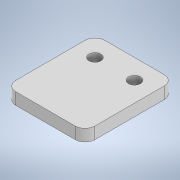
# Autodesk Inventor part: MagnetHolder_Special
Saved by Autodesk Inventor 2021 (Build 250183000, 183)
## iProperties
Created: 2021-12-05
Part Number: MagnetHolder_Special
Material: Generic
Document SubType Name: Modeling
Designer: Jorian Brusind
Density: 1 g/cm^3
Appearance: Default
Author: Jorian Brusind
Autodesk Inventor part; units mm, degrees
ref_plane "YZ Plane" through (0, 0, 0) normal (1, 0, 0) x (0, 1, 0)
ref_plane "XZ Plane" through (0, 0, 0) normal (0, 1, 0) x (-1, 0, 0)
ref_plane "XY Plane" through (0, 0, 0) normal (0, 0, 1) x (1, 0, 0)
sketch "Sketch20" plane through (0, 0, 0) normal (0, 1, 0) x (-1, 0, 0)
  line L0 (0, 0) -> (40, 0)
  line L1 (40, 0) -> (40, -45)
  line L2 (40, -45) -> (0, -45)
  line L3 (0, -45) -> (0, 0)
  line L4 (40, -45) -> (30, -45)
  line L5 (30, -45) -> (30, -35)
  line L6 (0, -45) -> (10, -45)
  line L7 (10, -45) -> (10, -35)
  circle A0 centre (30, -35) radius 3
  circle A1 centre (10, -35) radius 3
  dimension "d117" = 40
  dimension "d118" = 45
  dimension "d119" = 10
  dimension "d120" = 10
  dimension "d121" = 10
  dimension "d122" = 10
  dimension "d123" = 6
  dimension "d124" = 6
  constraints: 16 end point, 3 perpendicular, 2 centre point, 2 coincident, 2 parallel, 2 point on line, 1 horizontal
  measures "d117" distance of L1.end L2.end
  measures "d118" distance of L0.end L1.end
  measures "d119" distance of L1.end L4.end
  measures "d120" distance of L4.end L5.end
  measures "d121" distance of L2.end L6.end
  measures "d122" distance of L6.end L7.end
  measures "d123" diameter of A0
  measures "d124" diameter of A1
extrude "Extrusion20" add sketch "Sketch20" along normal blind 6
fillet "Fillet6" radius 5 4 edges at (0, 3, 0) (-40, 3, 0) (0, 3, -45) (-40, 3, -45)
body "Solid2"
